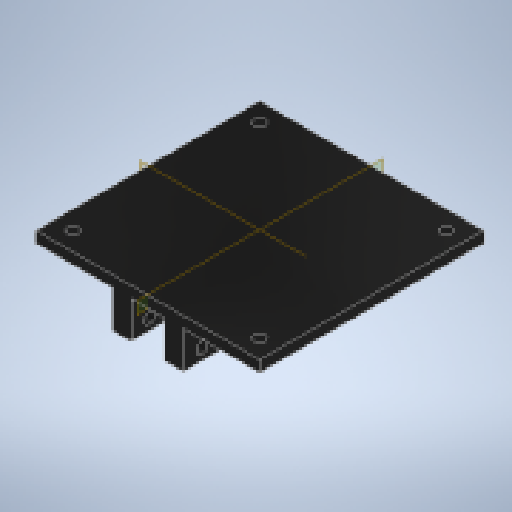
# Autodesk Inventor part: Slege_Mounting_Plate
Saved by Autodesk Inventor 2025.1 (Build 291241020, 241B)
## iProperties
Created: 2024-11-07
Part Number: Slege_Mounting_Plate
Material: Generic
Document SubType Name: Modeling
Designer: leon-
Density: 1 g/cm^3
Appearance: Smooth - Black
Author: leon-
Autodesk Inventor part; units mm, degrees
ref_plane "YZ Plane" through (0, 0, 0) normal (1, 0, 0) x (0, 1, 0)
ref_plane "XZ Plane" through (0, 0, 0) normal (0, 1, 0) x (-1, 0, 0)
ref_plane "XY Plane" through (0, 0, 0) normal (0, 0, 1) x (1, 0, 0)
sketch "Sketch1" plane through (0, 0, 0) normal (0, 1, 0) x (-1, 0, 0)
  line L0 (0, 0) -> (60, 0)
  line L1 (60, 0) -> (60, -60)
  line L2 (60, -60) -> (0, -60)
  line L3 (0, -60) -> (0, 0)
  dimension "d0" = 60
  dimension "d1" = 60
  constraints: 8 end point, 2 parallel, 1 horizontal, 1 perpendicular
  measures "d0" distance of L0.end L1.end
  measures "d1" distance of L1.end L2.end
extrude "Extrusion1" add sketch "Sketch1" along normal blind 3
sketch "Sketch2" plane through (0, 3, 0) normal (0, 1, 0) x (1, 0, 0)
  line L0 (-60, 0) -> (0, 0) projected
  line L1 (-60, 60) -> (-60, 0) projected
  point P0 (-55, 5)
  dimension "d4" = 5
  dimension "d5" = 5
  measures "d4" distance from line of L0 point (-55, 5)
  measures "d5" distance from line of L1 point (-55, 5)
hole "Hole1" at (-55, 3, -5) direction (0, -1, 0) diameter 3 end through all
ref_plane "Work Plane1" through (-30, 0, -60) normal (-1, 0, 0) x (0, 0, 1)
ref_plane "Work Plane2" through (-60, 0, -30) normal (0, 0, 1) x (1, 0, 0)
mirror "Mirror1" about plane through (-30, 0, -60) normal (-1, 0, 0) of "Hole1"
mirror "Mirror2" about plane through (-60, 0, -30) normal (0, 0, 1) of "Hole1", "Mirror1"
sketch "Sketch3" plane through (0, 0, 0) normal (0, -1, 0) x (1, 0, 0)
  line L0 (-39.5, 0) -> (-34.5, 0)
  line L1 (-34.5, 0) -> (-34.5, -60)
  line L2 (-34.5, -60) -> (-39.5, -60)
  line L3 (-39.5, -60) -> (-39.5, 0)
  line L4 (0, -60) -> (-60, -60) projected
  line L5 (-60, 0) -> (0, 0) projected
  line L6 (-30, -72) -> (-30, 12) projected
  dimension "d13" = 5
  dimension "d14" = 4.5
  constraints: 8 end point, 2 collinear, 2 parallel, 1 horizontal, 1 perpendicular
  measures "d13" distance between parallel lines of L3 L1
  measures "d14" distance between parallel lines of L6 L1
extrude "Extrusion2" add sketch "Sketch3" along normal blind 10 contours L0 L1 L2 L3
sketch "Sketch4" plane through (-34.5, 0, 0) normal (1, 0, 0) x (0, 0, -1)
  line L0 (0, 0) -> (0, -10) projected
  line L1 (60, 0) -> (60, -10) projected
  line L2 (0, 0) -> (60, 0) projected
  line L3 (60, -10) -> (0, -10) projected
  point P0 (5, -7)
  point P1 (55, -7)
  dimension "d17" = 5
  dimension "d18" = 5
  dimension "d20" = 3
  dimension "d21" = 3
  measures "d17" distance from line of L0 point (5, -7)
  measures "d18" distance from line of L1 point (55, -7)
  measures "d20" distance from line of L3 point (5, -7)
  measures "d21" distance from line of L3 point (55, -7)
hole "Hole2" at (-34.5, -7, -5) at (-34.5, -7, -55) direction (-1, 0, 0) diameter 3 end through all
mirror "Mirror3" about plane through (-30, 0, -60) normal (-1, 0, 0) of "Extrusion2", "Hole2"
equation "\"d4\" = d5"
equation "\"d18\" = d17"
body "Solid1"
